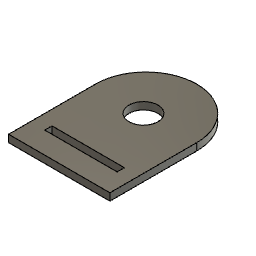
Assignment_01 (Autodesk Fusion 360 design; units mm, degrees)
Autodesk Fusion 360 part; units mm, degrees
box "BoxPrimitive1" add length 60 width 70 height 5 placed x (0, 0, -1) y (-1, 0, 0) z (0, 1, 0) at (10, 0, 10) makes body 1
move_body "Move2" bodies 1 to x (1, 0, 0) y (0, 1, 0) z (0, 0, 1) at (60, 0, 50)
box "BoxPrimitive3" add length 15 width 50 height 5 placed x (0, -1, 0) y (1, 0, 0) z (0, 0, 1) at (90, -40, 0) separate body makes body 2
move_body "Move3" bodies 2 to x (1, 0, 0) y (0, 1, 0) z (0, 0, 1) at (-80, 0, 20)
move_body "Move4" bodies 2 to x (1, 0, 0) y (0, 1, 0) z (0, 0, 1) at (0, 0, 12)
move_body "Move5" bodies 2 to x (1, 0, 0) y (0, 1, 0) z (0, 0, 1) at (-57, 0, 0)
extrude "Extrude1" add 1 faces at (-30.3333, -40, 33.6667) along direction (0, 1, 0) blind 30 on bodies 2 bodies 2
move_body "Move6" bodies 2 to x (1, 0, 0) y (0, 1, 0) z (0, 0, 1) at (50, 0, 0)
move_body "Move7" bodies 2 to x (1, 0, 0) y (0, 1, 0) z (0, 0, 1) at (-3, 0, 0)
move_body "Move8" bodies 2 to x (1, 0, 0) y (0, 1, 0) z (0, 0, 1) at (10, 0, 0)
move_body "Move9" bodies 2 to x (1, 0, 0) y (0, 1, 0) z (0, 0, 1) at (0, 0, 23)
move_body "Move10" bodies 2 to x (1, 0, 0) y (0, 1, 0) z (0, 0, 1) at (0, 0, -15)
cylinder "CylinderPrimitive1" add diameter 20 height 10 placed x (1, 0, 0) y (0, 0, -1) z (0, 1, 0) at (-15.8982, 0, -33.5833) separate body makes body 3
move_body "Move11" bodies 3 to x (1, 0, 0) y (0, 1, 0) z (0, 0, 1) at (50, 0, 10)
move_body "Move12" bodies 2 to x (1, 0, 0) y (0, 1, 0) z (0, 0, 1) at (0, 20, 0)
extrude "Extrude3" cut 1 faces at (26.6667, -35, 41.6667) along direction (0, 1, 0) blind 35 on bodies 2 bodies 2
move_body "Move13" bodies 3 to x (1, 0, 0) y (0, 1, 0) z (0, 0, 1) at (0, 0, 23.5)
box "BoxPrimitive4" add length 15 width 70 height 5 placed x (0, 0, 1) y (1, 0, 0) z (0, 1, 0) at (0, 0, -15) separate body makes body 4
move_face "MoveFace3" by (0, 0, -15) 1 faces at (23.3333, 1.6667, -15) on bodies 4
extrude "Extrude4" add 1 faces at (23.3333, 1.6667, -30) along direction (0, 0, -1) blind 5 on bodies 4 bodies 4
fillet "Fillet1" radius 35 1 edges at (0, 2.5, -35) on bodies 4
fillet "Fillet2" radius 35 1 edges at (70, 2.5, -35) on bodies 4
combine "Combine1" operation add target body 1 tool bodies 4
move_body "Move15" bodies 2 to x (1, 0, 0) y (0, 1, 0) z (0, 0, 1) at (0, -5, 0)
move_face "MoveFace4" by (0, 5, 0) 1 faces at (26.6667, -5, 41.6667) on bodies 2
move_body "Move16" bodies 3 to x (1, 0, 0) y (0, 1, 0) z (0, 0, 1) at (0, -5, 0)
move_face "MoveFace5" by (0, 5, 0) 1 faces at (32.4529, -5, -6.0465) on bodies 3
move_body "Move14" bodies 3 to x (1, 0, 0) y (0, 1, 0) z (0, 0, 1) at (0, 0, 1)
combine "Combine2" operation cut target body 1 tool bodies 3
combine "Combine3" operation cut target body 1 tool bodies 2
sketch "Sketch6" plane through (0, 0, 45) normal (0, 0, 1) x (1, 0, 0)
  line L0 (10, -55) -> (60, -55)
  line L1 (60, -55) -> (60, -10)
  line L2 (60, -10) -> (10, -10)
  line L3 (10, -10) -> (10, -55)
extrude "Extrude2" [suppressed]
moveface "MoveFace1" [suppressed]
moveface "MoveFace2" [suppressed]
boxprimitive "BoxPrimitive2" [suppressed]
move_body "Move1" [suppressed]
